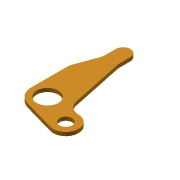
# Autodesk Inventor part: 3136 1133 81
Saved by Autodesk Inventor 2022 Beta2 (Build 260130000, 130) ContinuousBuild 0
## iProperties
Shininess: 64.0
Length Units: 11269
Angle Units: 11279
Time Units: 11290
Mass Units: 11283
Length Display Precision: 3
Angle Display Precision: 2
Compacted: True
Part Number: 3136 1133 81
Document SubType Name: Modeling
Created: 2003-04-13
Designer: Uffe Bak
Material: Steel, Mild
Density: 7.86 g/cm^3
Appearance: Brokk-Gul
Density: 0.0
Volumn: 0.0
Area: 0.0
PropertySet Name: Model Information
Control State: 0
Master: False
Checked Out: False
Author: Uffe Bak
Autodesk Inventor part; units mm, degrees
ref_plane "YZ Plane" through (0, 0, 0) normal (1, 0, 0) x (0, 1, 0)
ref_plane "XZ Plane" through (0, 0, 0) normal (0, 1, 0) x (-1, 0, 0)
ref_plane "XY Plane" through (0, 0, 0) normal (0, 0, 1) x (1, 0, 0)
sketch "Sketch1" plane through (0, 0, 0) normal (0, 0, 1) x (1, 0, 0)
  line L0 (-115.9793, -35.2742) -> (-115.9793, 64.2246)
  arc A0 (-113.8324, 76.2941) -> (-115.9793, 64.2246) centre (-80.9793, 64.2246) ccw
  line L1 (-113.8324, 76.2941) -> (-93.1262, 132.6563)
  arc A1 (-93.1262, 132.6563) -> (-90.9793, 144.7258) centre (-125.9793, 144.7258) ccw
  line L2 (-90.9793, 144.7258) -> (-90.9793, 174.7258)
  arc A2 (-50.9793, 174.7258) -> (-90.9793, 174.7258) centre (-70.9793, 174.7258) ccw
  line L3 (-50.9793, 174.7258) -> (-50.9793, 144.7258)
  arc A3 (-50.9793, 144.7258) -> (-50.222, 137.4844) centre (-15.9793, 144.7258) ccw
  line L4 (-50.222, 137.4844) -> (-19.622, -7.2156)
  arc A4 (-115.9793, -35.2742) -> (-83.2704, -78.5631) centre (-70.9793, -35.2742) ccw
  line L5 (-83.2704, -78.5631) -> (5.0609, -103.6433)
  arc A5 (5.0609, -103.6433) -> (14.6207, -34.9742) centre (14.6207, -69.9742) ccw
  arc A6 (-19.622, -7.2156) -> (14.6207, -34.9742) centre (14.6207, 0.0258) ccw
  circle A7 centre (-70.9793, -35.2742) radius 30
  circle A8 centre (14.6207, -69.9742) radius 17.5
  dimension "d0" = 20
  dimension "d1" = 210
  dimension "d4" = 85.6
  dimension "d5" = 34.7
  dimension "d7" = 35
  dimension "d8" = 35
  dimension "d9" = 35
  dimension "d10" = 35
  dimension "d11" = 45
  dimension "d12" = 35
  dimension "d13" = 100
  dimension "d15" = 35
  dimension "d16" = 60
  dimension "d17" = 180
  dimension "d18" = 180
  constraints: 14 point on circle, 13 tangent, 12 end point, 9 centre point, 3 coincident, 2 concentric, 2 parallel, 2 vertical alignment, 1 vertical, 1 other
  measures "d0" radius of A2
  measures "d1" distance of A4.centre A2.centre
  measures "d4" horizontal distance of A4.centre A5.centre
  measures "d5" vertical distance of A4.centre A5.centre
  measures "d7" radius of A1
  measures "d8" radius of A0
  measures "d9" radius of A3
  measures "d10" radius of A5
  measures "d11" radius of A4
  measures "d12" radius of A6
  measures "d13" distance of A0.centre A4.centre
  measures "d15" diameter of A8
  measures "d16" diameter of A7
  measures "d17" vertical distance of A3.centre A4.centre
  measures "d18" vertical distance of A1.centre A4.centre
extrude "Extrusion1" add sketch "Sketch1" along normal blind 10
equation "\"d8\" = d7"
equation "\"d9\" = d7"
equation "\"d10\" = d9"
body "Solid1"
